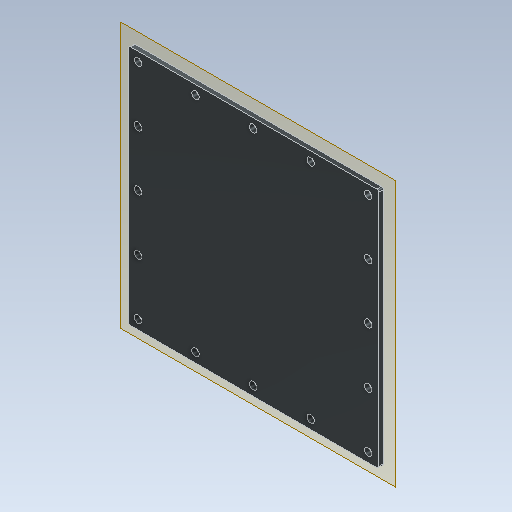
# Autodesk Inventor part: Крышка водяной рубашки
Saved by Autodesk Inventor 2021 (Build 250183000, 183)
## iProperties
Created: 2020-12-12
Part Number: Крышка водяной рубашки
Material: Чугун, серый
Document SubType Name: Modeling
Designer: Тимоха
Mass: 2474.01 g
Surface Area: 1456.92 cm^2
Volume: 346.015 cm^3
Density: 7.15 g/cm^3
Appearance: Чугун серый
Author: Тимоха
Autodesk Inventor part; units mm, degrees
ref_plane "YZ Plane" through (0, 0, 0) normal (1, 0, 0) x (0, 1, 0)
ref_plane "XZ Plane" through (0, 0, 0) normal (0, 1, 0) x (-1, 0, 0)
ref_plane "XY Plane" through (0, 0, 0) normal (0, 0, 1) x (1, 0, 0)
ref_plane "РабПлоскость1" through (0, 0, 0) normal (0, 0, 1) x (1, 0, 0)
sketch "Эскиз1" plane through (0, 0, 0) normal (0, 0, 1) x (1, 0, 0)
  line L0 (-134.636, 128) -> (-134.636, -128) projected
  arc A0 (-134.636, -128) -> (-132.636, -130) centre (-132.636, -128) ccw projected
  line L1 (-132.636, -130) -> (132.636, -130) projected
  arc A1 (132.636, -130) -> (134.636, -128) centre (132.636, -128) ccw projected
  line L2 (134.636, -128) -> (134.636, 128) projected
  arc A2 (134.636, 128) -> (132.636, 130) centre (132.636, 128) ccw projected
  line L3 (132.636, 130) -> (-132.636, 130) projected
  arc A3 (-132.636, 130) -> (-134.636, 128) centre (-132.636, 128) ccw projected
  circle A4 centre (-124.636, 120) radius 4 projected
  circle A5 centre (-0.636, 120) radius 4 projected
  circle A6 centre (123.364, 120) radius 4 projected
  circle A7 centre (123.364, 60) radius 4 projected
  circle A8 centre (123.364, 0) radius 4 projected
  circle A9 centre (-124.636, -60) radius 4 projected
  circle A10 centre (123.364, -60) radius 4 projected
  circle A11 centre (-124.636, -120) radius 4 projected
  circle A12 centre (-62.636, -120) radius 4 projected
  circle A13 centre (-0.636, -120) radius 4 projected
  circle A14 centre (61.364, -120) radius 4 projected
  circle A15 centre (123.364, -120) radius 4 projected
  circle A16 centre (-124.636, 0) radius 4 projected
  circle A17 centre (-124.636, 60) radius 4 projected
  circle A18 centre (61.364, 120) radius 4 projected
  circle A19 centre (-62.636, 120) radius 4 projected
  line L4 (115.364, 110) -> (115.364, -110) projected
  line L5 (115.364, -110) -> (-114.636, -110) projected
  line L6 (-114.636, -110) -> (-114.636, 110) projected
  line L7 (-114.636, 110) -> (115.364, 110) projected
  point P0 (0, 0)
extrude "Выдавливание1" add sketch "Эскиз1" along normal blind 5 contours A3 L3 A2 L2 A1 L1 A0 L0 | L4 L5 L6 L7
